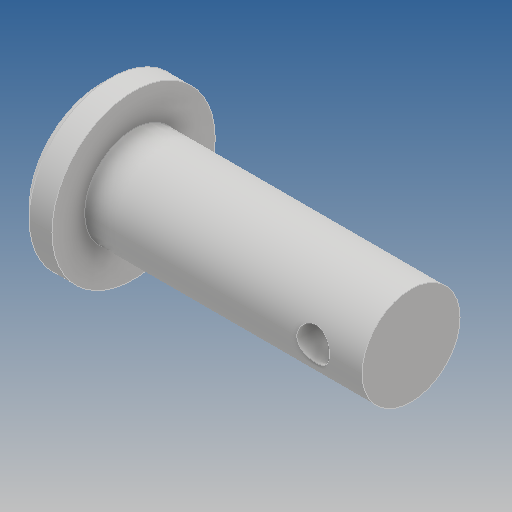
# Autodesk Inventor part: Bolzen
Saved by Autodesk Inventor 2018 (Build 220112000, 112)
## iProperties
Created: 2018-10-23
Part Number: Bolzen
Material: Generisch
Document SubType Name: Modeling
Designer: M.Knabel
Density: 1 g/cm^3
Appearance: Vorgabe
Mass: 0.0767162 g
Surface Area: 1.39763 cm^2
Volume: 0.0767162 cm^3
Author: M.Knabel
Autodesk Inventor part; units mm, degrees
ref_plane "YZ Plane" through (0, 0, 0) normal (1, 0, 0) x (0, 1, 0)
ref_plane "XY Plane" through (0, 0, 0) normal (0, 0, 1) x (1, 0, 0)
sketch "Skizze1" plane through (0, 0, 0) normal (0, 0, 1) x (1, 0, 0)
  line L0 (0, -0.5) -> (0, 3) projected
  line L1 (-1.9, 0) -> (11.4, 0) projected
  line L2 (0, 0) -> (0, 2.5)
  line L3 (1, 2.5) -> (1, 1.5)
  line L4 (1, 1.5) -> (9.5, 1.5)
  line L5 (9.5, 1.5) -> (9.5, 0)
  line L6 (0, 0) -> (9.5, 0)
  line L7 (0, 2.5) -> (1, 2.5)
  dimension "d0" = 5
  dimension "d1" = 3
  dimension "d2" = 9.5
  dimension "d3" = 8.5
  constraints: 12 end point, 2 parallel, 2 point on line, 1 collinear, 1 perpendicular, 1 vertical
  measures "d0" diameter of L7 L1
  measures "d1" diameter of L4 L1
  measures "d2" distance between parallel lines of L5 L0
  measures "d3" distance between parallel lines of L5 L3
revolve "Umdrehung1" add sketch "Skizze1" angle 360 about axis through (-10, 0, 0) along (1, 0, 0)
chamfer "Fase1" distance 0.3 angle 45 1 edges at (0, -2.5, 0)
ref_plane "Arbeitsebene1" through (5.25, 1.5, 0) normal (0, 1, 0) x (-1, 0, 0)
sketch "Skizze2" plane through (5.25, 1.5, 0) normal (0, 1, 0) x (-1, 0, 0)
  line L0 (4.25, 1.5) -> (4.25, -1.5) projected
  line L1 (-4.25, 1.5) -> (-4.25, -1.5) projected
  line L2 (4.25, 1.5) -> (4.25, -1.5) projected
  line L3 (-4.25, 1.5) -> (-4.25, -1.5) projected
  line L4 (4.25, 1.5) -> (-4.25, 1.5) projected
  line L5 (4.25, -1.5) -> (-4.25, -1.5) projected
  point P0 (5.25, 0)
  point P1 (-2.75, 0)
  dimension "d8" = 1.5
  dimension "d9" = 1.5
  measures "d8" distance from line of point (-2.75, 0) L1
  measures "d9" distance from line of L5 point (-2.75, 0)
hole "Bohrung1" at (8, 1.5, 0) direction (0, -1, 0) diameter 1 end through all
